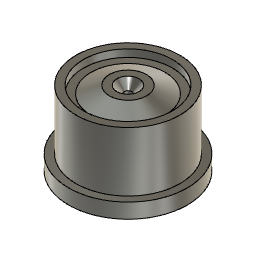
Чистики (Autodesk Fusion 360 design; units mm, degrees)
Autodesk Fusion 360 part; units mm, degrees
sketch "Sketch1" plane through (0, 0, 0) normal (0, 0, 1) x (1, 0, 0)
  circle A0 centre (30, 30) radius 7
  dimension "d1" = 14
  measures "d1" diameter of A0
extrude "Extrude1" add sketch "Sketch1" along normal blind 8
sketch "Sketch2" plane through (0, 0, 0) normal (0, 0, -1) x (1, 0, 0)
  circle A0 centre (30, -30) radius 7
  circle A1 centre (30, -30) radius 8
  dimension "d4" = 16
  constraint concentric A0 A1
  measures "d4" diameter of A1
extrude "Extrude2" add sketch "Sketch2" along normal blind 2 contours A0 | A1
sketch "Sketch3" plane through (0, 0, 8) normal (0, 0, 1) x (-1, 0, 0)
  circle A0 centre (-30, -30) radius 7
  circle A1 centre (-30, -30) radius 2.5
  circle A2 centre (-30, -30) radius 1.5
  circle A3 centre (-30, -30) radius 6
  circle A4 centre (-30, -30) radius 0.5
  circle A5 centre (-30, -30) radius 5
  dimension "d7" = 5
  dimension "d8" = 3
  dimension "d9" = 12
  dimension "d10" = 1
  dimension "d13" = 10
  constraint concentric A0 A1
  constraint concentric A1 A2
  constraint concentric A1 A3
  constraint concentric A1 A4
  constraint concentric A4 A5
  measures "d7" diameter of A1
  measures "d8" diameter of A2
  measures "d9" diameter of A3
  measures "d10" diameter of A4
  measures "d13" diameter of A5
extrude "Extrude3" cut sketch "Sketch3" against normal blind 16 contours A4
extrude "Extrude4" cut sketch "Sketch3" against normal blind 1 contours A3
chamfer "Chamfer1" distance 2.5 distance2 1 1 edges at (34.6616, 31.8081, 8) measured on face at (26.5186, 30.2484, 8)
chamfer "Chamfer2" distance 1 distance2 1 1 edges at (30.4662, 29.8192, 8) measured on face at (28.1756, 30.1242, 8)
sketch "Sketch4" plane through (0, 0, -2) normal (0, 0, -1) x (1, 0, 0)
  circle A0 centre (30, -30) radius 0.5
  circle A1 centre (30, -30) radius 8
  circle A2 centre (30, -30) radius 5
  dimension "d20" = 10
  constraint concentric A0 A2
  measures "d20" diameter of A2
chamfer "Chamfer3" distance 4.5 distance2 8.5 1 edges at (30.4662, 30.1808, -2) measured on face at (35.4684, 30.4223, -2)
